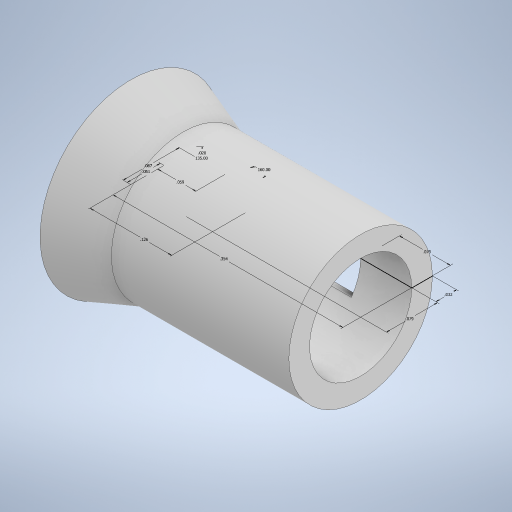
# Autodesk Inventor part: collimator
Saved by Autodesk Inventor 2024 (Build 280153000, 153)
## iProperties
Created: 2024-10-31
Part Number: collimator
Material: Generic
Document SubType Name: Modeling
Designer: Williamow
Density: 1 g/cm^3
Appearance: Default
Author: Williamow
Autodesk Inventor part; units mm, degrees
ref_plane "YZ Plane" through (0, 0, 0) normal (1, 0, 0) x (0, 1, 0)
ref_plane "XZ Plane" through (0, 0, 0) normal (0, 1, 0) x (-1, 0, 0)
ref_plane "XY Plane" through (0, 0, 0) normal (0, 0, 1) x (1, 0, 0)
sketch "Sketch1" plane through (0, 0, 0) normal (0, 1, 0) x (-1, 0, 0)
  line L0 (0, 0) -> (-2.1541, 0)
  line L1 (0, -2.5536) -> (-0.3536, -2.2)
  line L2 (-1.5, -2.2) -> (-2.0495, -2)
  line L3 (-2.0495, -2) -> (-9, -2)
  line L4 (-9, -2) -> (-9, -2.81)
  line L5 (-9, -2.81) -> (-2.0495, -2.81)
  line L6 (-2.0495, -2.81) -> (0, -3.556)
  line L7 (0, -3.556) -> (0, -2.5536)
  line L8 (-2.0495, -2) -> (-2.0495, -2.81)
  line L9 (-7, -2) -> (-7, -2.81)
  line L10 (-0.3536, -2.2) -> (-1.5, -2.2)
  line L11 (0, -1.3) -> (-3.2, -1.3)
  point P0 (0, 0)
  dimension "d1" = 2
  dimension "d2" = 160
  dimension "d3" = 0.81
  dimension "d4" = 9
  dimension "d6" = 2
  dimension "d9" = 2.2
  dimension "d10" = 0.5
  dimension "d11" = 135
  dimension "d12" = 1.5
  dimension "d13" = 3.2
  dimension "d14" = 1.3
  constraints: 24 end point, 3 horizontal, 3 perpendicular, 3 vertical alignment, 2 parallel, 2 point on line, 2 vertical, 1 coincident
  measures "d1" distance between parallel lines of L0 L3
  measures "d2" angle of L6 L5
  measures "d3" distance of L3.end L4.end
  measures "d4" horizontal distance of point (0, 0) L3.end
  measures "d6" distance between parallel lines of L4 L9
  measures "d9" distance from line of point (0, 0) L10
  measures "d10" distance of L1.start L1.end
  measures "d11" angle of L10 L1
  measures "d12" horizontal distance of point (0, 0) L2.start
  measures "d13" distance of L11.start L11.end
  measures "d14" distance between parallel lines of L0 L11
revolve "Revolution1" add sketch "Sketch1" angle 360 about axis through (0, 0, 0) along (1, 0, 0)
revolve "Revolution2" cut sketch "Sketch1" angle 70 mid plane about axis through (0, 0, 0) along (1, 0, 0) contours L5 L9 L3 L8
body "Solid1"
